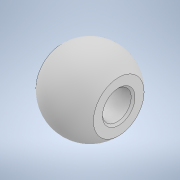
# Autodesk Inventor part: eye_bearing_1
Saved by Autodesk Inventor 2020 (Build 240168000, 168)
## iProperties
Created: 2020-01-21
Part Number: eye_bearing_1
Material: Generic
Document SubType Name: Modeling
Designer: psrobotics
Density: 1 g/cm^3
Appearance: Default
Author: psrobotics
Autodesk Inventor part; units mm, degrees
ref_plane "YZ Plane" through (0, 0, 0) normal (1, 0, 0) x (0, 1, 0)
ref_plane "XZ Plane" through (0, 0, 0) normal (0, 1, 0) x (-1, 0, 0)
ref_plane "XY Plane" through (0, 0, 0) normal (0, 0, 1) x (1, 0, 0)
sketch "Sketch1" plane through (0, 0, 0) normal (0, 1, 0) x (-1, 0, 0)
  circle A0 centre (0, 0) radius 4
  line L0 (0, 0) -> (4, 0)
  line L1 (0, 0) -> (-4, 0)
  dimension "d0" = 8
  constraints: 4 end point, 2 point on circle, 1 centre point, 1 coincident, 1 horizontal, 1 point on line
  measures "d0" diameter of A0
revolve "Revolution1" add sketch "Sketch1" angle 360 about axis through (0, 0, 0) along (1, 0, 0) picked at (2.6279, -0.3191) contours A0 L1 L0
sketch "Sketch2" plane through (0, 0, 0) normal (0, 1, 0) x (-1, 0, 0)
  circle A0 centre (0, 0) radius 4 projected
  line L0 (0, 0) -> (3, 0)
  line L1 (0, 0) -> (-3, 0)
  line L2 (3, 0) -> (3, -2.6458)
  line L3 (3, 0) -> (3, 2.6458)
  line L4 (-3, 0) -> (-3, -2.6458)
  line L5 (-3, 0) -> (-3, 2.6458)
  dimension "d2" = 3
  dimension "d3" = 3
  constraints: 12 end point, 4 point on circle, 2 horizontal, 2 point on line, 1 parallel, 1 vertical
  measures "d2" distance of L0.start L0.end
  measures "d3" distance of L0.start L1.end
extrude "Extrusion1" cut sketch "Sketch2" along normal mid plane 10 contours A0 L2 L3 | L5 L4 A0
sketch "Sketch3" plane through (3, 0, 0) normal (1, 0, 0) x (0, 0, -1)
  circle A0 centre (0, 0) radius 2.6458 projected
  circle A1 centre (0, 0) radius 1.5
  dimension "d6" = 3
  constraints: 1 centre point, 1 coincident
  measures "d6" diameter of A1
extrude "Extrusion2" cut sketch "Sketch3" against normal blind 10 contours A1
chamfer "Chamfer1" distance 0.2 angle 45 2 edges at (3, 0, 1.5) (-3, 0, 1.5)
body "Solid1"
